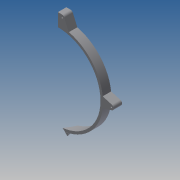
# Autodesk Inventor part: wheel_rim_mold_B
Saved by Autodesk Inventor 2016 (Build 200138000, 138)
## iProperties
Created: 2014-06-11
Part Number: wheel_rim_mold_B
Material: Générique
Document SubType Name: Modeling
Designer: Yann
Density: 1 g/cm^3
Appearance: Par défaut
Mass: 582.103 g
Surface Area: 940.952 cm^2
Volume: 582.103 cm^3
Author: Yann
Autodesk Inventor part; units mm, degrees
ref_plane "YZ Plane" through (0, 0, 0) normal (1, 0, 0) x (0, 1, 0)
ref_plane "XZ Plane" through (0, 0, 0) normal (0, 1, 0) x (-1, 0, 0)
ref_plane "XY Plane" through (0, 0, 0) normal (0, 0, 1) x (1, 0, 0)
sketch "Esquisse1" plane through (0, 0, 0) normal (0, 0, 1) x (1, 0, 0)
  line L0 (-215.2, 20) -> (-215.2, -20)
  line L1 (-203.2, -20) -> (-203.2, 20)
  line L2 (-203.2, -20) -> (-215.2, -20)
  line L3 (-203.2, 20) -> (-215.2, 20)
  line L4 (0, -28.064) -> (0, 28.384) projected
  line L5 (-301.28, 0) -> (301.28, 0) construction
  line L6 (-215.2, 20.32) -> (215.2, 20.32) construction
  line L7 (203.2, 18.32) -> (-203.2, 18.32) construction
  point P0 (0, 0)
  dimension "d0" = 0
  dimension "d8" = 40
  constraints: 8 end point, 6 point on line, 4 vertical, 3 horizontal, 9 other
  measures "d8" distance of L0.start L0.end
revolve "Révolution1" add sketch "Esquisse1" angle 360 about axis through (0, -10, 0) along (0, 1, 0)
sketch "Esquisse2" plane through (0, 0, 0) normal (0, 1, 0) x (-1, 0, 0)
  arc A0 (130.8148, 194.4544) -> (-130.8148, 194.4544) centre (0, 63.6396) ccw construction
  line L0 (-194.4544, 130.8148) -> (-130.8148, 194.4544) construction
  arc A1 (-194.4544, 130.8148) -> (-194.4544, -130.8148) centre (-63.6396, 0) ccw construction
  line L1 (-130.8148, -194.4544) -> (-194.4544, -130.8148) construction
  arc A2 (-130.8148, -194.4544) -> (130.8148, -194.4544) centre (0, -63.6396) ccw construction
  line L2 (194.4544, -130.8148) -> (130.8148, -194.4544) construction
  arc A3 (194.4544, -130.8148) -> (194.4544, 130.8148) centre (63.6396, 0) ccw construction
  line L3 (130.8148, 194.4544) -> (194.4544, 130.8148) construction
  circle A4 centre (10.375, -17.97) radius 2.5 projected
  circle A5 centre (-10.375, -17.97) radius 2.5 projected
  circle A6 centre (-20.75, 0) radius 2.5 projected
  circle A7 centre (-10.375, 17.97) radius 2.5 projected
  circle A8 centre (10.375, 17.97) radius 2.5 projected
  circle A9 centre (20.75, 0) radius 2.5 projected
  circle A10 centre (-20, 253.412) radius 4
  circle A11 centre (20, 253.412) radius 4
  circle A12 centre (-254.2, 0) radius 4
  circle A13 centre (254.2, 0) radius 4
  circle A14 centre (0, 0) radius 215.2 projected
  circle A15 centre (0, 0) radius 215.2 construction
  line L4 (-52.3712, 208.7302) -> (-31.0163, 258.1703)
  arc A16 (-20, 265.412) -> (-31.0163, 258.1703) centre (-20, 253.412) ccw
  line L5 (0, -397.3869) -> (0, 397.3869) construction
  line L6 (-397.3869, 0) -> (397.3869, 0) construction
  line L7 (-20, 265.412) -> (0, 265.412)
  arc A17 (0, 215.2) -> (-52.3712, 208.7302) centre (0, 0) ccw
  line L8 (0, 215.2) -> (0, 265.412)
  line L9 (52.3712, 208.7302) -> (31.0163, 258.1703)
  arc A18 (31.0163, 258.1703) -> (20, 265.412) centre (20, 253.412) ccw
  line L10 (20, 265.412) -> (0, 265.412)
  arc A19 (52.3712, 208.7302) -> (0, 215.2) centre (0, 0) ccw
  circle A20 centre (-20, -253.412) radius 4
  line L11 (-52.3712, -208.7302) -> (-31.0163, -258.1703)
  arc A21 (-31.0163, -258.1703) -> (-20, -265.412) centre (-20, -253.412) ccw
  line L12 (-20, -265.412) -> (0, -265.412)
  arc A22 (-52.3712, -208.7302) -> (0, -215.2) centre (0, 0) ccw
  line L13 (0, -215.2) -> (0, -265.412)
  line L14 (52.3712, -208.7302) -> (31.0163, -258.1703)
  arc A23 (20, -265.412) -> (31.0163, -258.1703) centre (20, -253.412) ccw
  line L15 (20, -265.412) -> (0, -265.412)
  arc A24 (0, -215.2) -> (52.3712, -208.7302) centre (0, 0) ccw
  line L16 (-213.8059, -24.4559) -> (-257.6022, -11.5076)
  arc A25 (-215.2, 0) -> (-213.8059, -24.4559) centre (0, 0) ccw
  line L17 (-213.8059, 24.4559) -> (-257.6022, 11.5076)
  arc A26 (-257.6022, 11.5076) -> (-257.6022, -11.5076) centre (-254.2, 0) ccw
  arc A27 (-213.8059, 24.4559) -> (-215.2, 0) centre (0, 0) ccw
  line L18 (213.8059, -24.4559) -> (257.6022, -11.5076)
  arc A28 (257.6022, -11.5076) -> (260.1568, -10.4171) centre (254.2, 0) ccw
  arc A29 (213.8059, -24.4559) -> (215.2, 0) centre (0, 0) ccw
  arc A30 (260.1568, -10.4171) -> (257.6022, 11.5076) centre (254.2, 0) ccw
  line L19 (213.8059, 24.4559) -> (257.6022, 11.5076)
  arc A31 (215.2, 0) -> (213.8059, 24.4559) centre (0, 0) ccw
  circle A32 centre (254.2, 0) radius 4 projected
  circle A33 centre (-254.2, 0) radius 4 projected
  circle A34 centre (-20, -253.412) radius 4 projected
  circle A35 centre (20, 253.412) radius 4 projected
  circle A36 centre (-20, 253.412) radius 4 projected
  line L20 (-254.5584, 70.7107) -> (-70.7107, 254.5584) projected
  arc A37 (70.7107, 254.5584) -> (-70.7107, 254.5584) centre (0, 183.8478) ccw projected
  line L21 (70.7107, 254.5584) -> (254.5584, 70.7107) projected
  arc A38 (254.5584, -70.7107) -> (254.5584, 70.7107) centre (183.8478, 0) ccw projected
  line L22 (254.5584, -70.7107) -> (70.7107, -254.5584) projected
  arc A39 (-70.7107, -254.5584) -> (70.7107, -254.5584) centre (0, -183.8478) ccw projected
  line L23 (-70.7107, -254.5584) -> (-254.5584, -70.7107) projected
  arc A40 (-254.5584, 70.7107) -> (-254.5584, -70.7107) centre (-183.8478, 0) ccw projected
  circle A41 centre (20, -253.412) radius 4 projected
  circle A42 centre (20, -253.412) radius 4
  dimension "d2" = 8
  dimension "d9" = 8
  dimension "d10" = 8
  constraints: 34 point on circle, 28 end point, 22 symmetric about line, 20 centre point, 10 coincident, 5 tangent, 2 collinear, 2 point on line, 1 concentric, 11 other
  measures "d2" radial gap between concentric circles of A16 A10
  measures "d9" diameter of A10
  measures "d10" radial gap between concentric circles of A26 A33
ref_plane "Plan de construction1" through (-292.132, 25.32, -292.132) normal (0, -1, 0) x (1, 0, 0)
ref_plane "Plan de construction2" through (-215.2, 20.32, -215.2) normal (0, -1, 0) x (1, 0, 0)
extrude "Extrusion1" add sketch "Esquisse2" along normal mid plane 40.5 contours A14 L19 A30 A28 L18 | A14 L8 L10 A18 L9 | L14 A23 L15 L13 A14 | A14 L4 A16 L7 L8 | L13 L12 A21 L11 A14 | A14 L16 A26 L17
split "Scission1" plane through (0, 0, 0) removes the side toward (-1, 0, 0)
